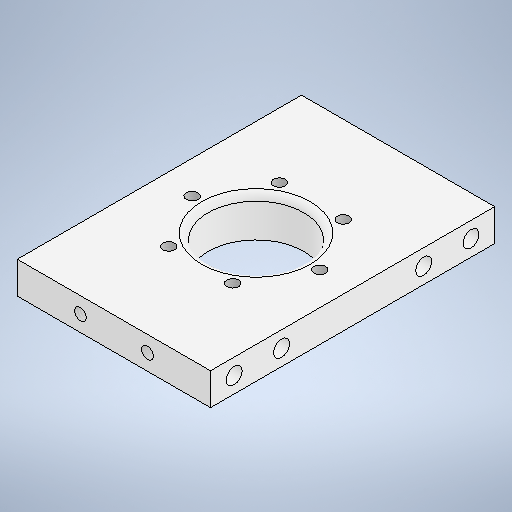
# Autodesk Inventor part: joint3_base2
Saved by Autodesk Inventor 2025.3 (Build 293356030, 356C)
## iProperties
Created: 2025-11-25
Part Number: joint3_base2
Material: PLA filament
Document SubType Name: Modeling
Designer: MSI
Mass: 55.5372 g
Surface Area: 164.624 cm^2
Volume: 46.281 cm^3
Density: 1.2 g/cm^3
Appearance: 일반
Author: MSI
Autodesk Inventor part; units mm, degrees
ref_plane "YZ Plane" through (0, 0, 0) normal (1, 0, 0) x (0, 1, 0)
ref_plane "XZ Plane" through (0, 0, 0) normal (0, 1, 0) x (-1, 0, 0)
ref_plane "XY Plane" through (0, 0, 0) normal (0, 0, 1) x (1, 0, 0)
sketch "스케치1" plane through (0, 0, 0) normal (0, 1, 0) x (-1, 0, 0)
  line L0 (107, -50) -> (-107, -50)
  line L1 (-107, -50) -> (-107, 50)
  line L2 (-107, 50) -> (107, 50)
  line L3 (107, 50) -> (107, -50)
  line L4 (107, -50) -> (-107, 50) construction
  line L5 (-107, -50) -> (107, 50) construction
  point P0 (0, 0)
  dimension "d0" = 214
  dimension "d1" = 100
  constraints: 12 end point, 2 midpoint, 2 parallel, 1 horizontal, 1 perpendicular
  measures "d0" distance of L1.end L2.end
  measures "d1" distance of L0.end L1.end
extrude "돌출1" add sketch "스케치1" along normal mid plane 10
sketch "스케치2" plane through (0, 5, 0) normal (0, 1, 0) x (1, 0, 0)
  point P0 (0, 0)
hole "구멍1" at (0, 5, 0) direction (0, -1, 0) diameter 30 end through all
fillet "모깎기2" radius 2 1 edges at (0, 5, -15)
sketch "스케치3" plane through (0, 5, 0) normal (0, 1, 0) x (1, 0, 0)
  line L0 (-107, 50) -> (-107, -50) projected
  line L1 (-107, 30) -> (-81.5, 30)
  line L2 (-81.5, 30) -> (-81.5, -30)
  line L3 (-81.5, -30) -> (-107, -30)
  line L4 (-107, -30) -> (-107, 30)
  line L5 (107, 50) -> (-107, 50) projected
  point P0 (0, 0)
  point P1 (-107, 0)
  dimension "d13" = 25.5
  dimension "d14" = 20
  constraints: 8 end point, 2 midpoint, 2 parallel, 1 horizontal, 1 perpendicular, 1 point on line
  measures "d13" distance of L2.end L3.end
  measures "d14" distance between parallel lines of L5 L1
extrude "돌출2" cut sketch "스케치3" against normal through all
sketch "스케치4" plane through (-81.5, 5, -30) normal (-1, 0, 0) x (0, 0, 1)
  line L0 (7, -5) -> (53, -5) construction
  point P0 (30, -5)
  point P1 (30, -5)
  point P2 (22.3333, -5)
  point P3 (37.6667, -5)
  dimension "d20" = 15.3333
  dimension "d21" = 15.3333
  dimension "d22" = 46
  constraints: 3 coincident, 2 end point, 2 point on line, 1 horizontal, 1 midpoint
  measures "d20" distance of point (22.333, -5) point (7, -5)
  measures "d21" distance of point (37.667, -5) point (53, -5)
  measures "d22" distance of L0.start L0.end
hole "구멍2" at (-81.5, 0, -23) at (-81.5, 0, -7.6667) at (-81.5, 0, 7.6667) at (-81.5, 0, 23) direction (1, 0, 0) diameter 3.6881 depth 12 tip angle 118 thread size "M4.5x0.75" class "6H" standard "ISO Metric profile"
sketch "스케치5" plane through (0, -5, 0) normal (0, -1, 0) x (1, 0, 0)
  line L0 (-100.75, -40) -> (-88.25, -40) construction
  line L1 (-88.25, -40) -> (-88.25, 40) construction
  line L2 (-88.25, 40) -> (-100.75, 40) construction
  line L3 (-100.75, 40) -> (-100.75, -40) construction
  line L4 (-107, -50) -> (107, -50) projected
  line L5 (-107, -30) -> (-107, -50) projected
  line L6 (107, 50) -> (-107, 50) projected
  point P0 (0, 0)
  dimension "d30" = 10
  dimension "d31" = 6.25
  dimension "d32" = 12.5
  dimension "d33" = 10
  constraints: 8 end point, 4 coincident, 2 parallel, 1 horizontal, 1 perpendicular
  measures "d30" distance between parallel lines of L0 L4
  measures "d31" distance between parallel lines of L3 L5
  measures "d32" distance of L0.start L0.end
  measures "d33" distance between parallel lines of L6 L2
hole "구멍3" at (-100.75, -5, -40) at (-88.25, -5, -40) at (-88.25, -5, 40) at (-100.75, -5, 40) direction (0, 1, 0) diameter 4.5 end through all counterbore diameter 8 counterbore depth 4.4 clearance for "Socket Head Cap Screw ISO 4762" size "M4" standard "ISO"
mirror "미러1" about plane through (0, 0, 0) normal (1, 0, 0) of "돌출2", "구멍2", "구멍3"
sketch "스케치6" plane through (0, -5, 0) normal (0, -1, 0) x (1, 0, 0)
  circle A0 centre (0, 0) radius 15 projected
  line L0 (25.9808, 0) -> (12.9904, -22.5)
  line L1 (12.9904, -22.5) -> (-12.9904, -22.5)
  line L2 (-12.9904, -22.5) -> (-25.9808, 0)
  line L3 (-25.9808, 0) -> (-12.9904, 22.5)
  line L4 (-12.9904, 22.5) -> (12.9904, 22.5)
  line L5 (12.9904, 22.5) -> (25.9808, 0)
  dimension "d41" = 45
  constraints: 12 end point, 1 coincident, 1 horizontal, 13 other
  measures "d41" distance between parallel lines of L1 L4
extrude "돌출3" add sketch "스케치6" along normal blind 2.5
sketch "스케치7" plane through (0, 5, 0) normal (0, 1, 0) x (1, 0, 0)
  line L0 (0, 0) -> (-20, 0) construction
  dimension "d44" = 20
  constraints: 2 end point, 1 horizontal
  measures "d44" distance of L0.start L0.end
hole "구멍4" at (-20, 5, 0) direction (0, -1, 0) diameter 3.6881 end through all thread size "M4.5x0.75" class "6H" standard "ISO Metric profile"
pattern_circular "원형 패턴1" count 6 over 360 about axis through (0, 3, 0) along (0, -1, 0) of "구멍4"
sketch "스케치8" plane through (0, -5, 0) normal (0, -1, 0) x (1, 0, 0)
  line L0 (-53.279, 16.5) -> (-38.279, 16.5) construction
  line L1 (-38.279, 16.5) -> (-38.279, -16.5) construction
  line L2 (-38.279, -16.5) -> (-53.279, -16.5) construction
  line L3 (-53.279, -16.5) -> (-53.279, 16.5) construction
  line L4 (-53.279, 16.5) -> (-38.279, -16.5) construction
  line L5 (-38.279, 16.5) -> (-53.279, -16.5) construction
  line L6 (-107, -50) -> (107, -50) projected
  line L7 (0, -50) -> (0, 50) construction
  line L8 (107, 50) -> (-107, 50) projected
  line L9 (-50.279, -13.5) -> (-41.279, -13.5) construction
  line L10 (-41.279, -13.5) -> (-41.279, 13.5) construction
  line L11 (-41.279, 13.5) -> (-50.279, 13.5) construction
  line L12 (-50.279, 13.5) -> (-50.279, -13.5) construction
  line L13 (53.279, 16.5) -> (38.279, 16.5) construction
  line L14 (38.279, 16.5) -> (38.279, -16.5) construction
  line L15 (38.279, -16.5) -> (53.279, -16.5) construction
  line L16 (53.279, -16.5) -> (53.279, 16.5) construction
  line L17 (53.279, 16.5) -> (38.279, -16.5) construction
  line L18 (38.279, 16.5) -> (53.279, -16.5) construction
  line L19 (50.279, -13.5) -> (41.279, -13.5) construction
  line L20 (41.279, -13.5) -> (41.279, 13.5) construction
  line L21 (41.279, 13.5) -> (50.279, 13.5) construction
  line L22 (50.279, 13.5) -> (50.279, -13.5) construction
  point P0 (0, 0)
  point P1 (-45.779, 0)
  point P2 (45.779, 0)
  dimension "d55" = 33
  dimension "d56" = 15
  dimension "d57" = 38.279
  dimension "d58" = 3
  constraints: 42 end point, 13 symmetric about line, 8 coincident, 4 midpoint, 4 parallel, 2 perpendicular, 1 horizontal, 1 horizontal alignment, 3 other
  measures "d55" distance of L2.end L0.start
  measures "d56" distance of L1.end L2.end
  measures "d57" distance between parallel lines of L7 L1
  measures "d58" distance between parallel lines of L2 L9
hole "구멍5" at (-50.279, -5, 13.5) at (-41.279, -5, 13.5) at (-41.279, -5, -13.5) at (-50.279, -5, -13.5) at (50.279, -5, -13.5) at (41.279, -5, -13.5) at (41.279, -5, 13.5) at (50.279, -5, 13.5) direction (0, 1, 0) diameter 4.5 end through all counterbore diameter 8 counterbore depth 4.6 clearance for "Socket Head Cap Screw ISO 4762" size "M4" standard "ISO"
chamfer "모따기1" distance 1 angle 45 4 edges at (107, 0, -30) (107, 0, 30) (-107, 0, -30) (-107, 0, 30)
fillet "모깎기1" radius 3 10 edges at (107, 0, 50) (107, 0, -50) (-107, 0, -50) (-107, 0, 50) (-12.9904, -6.25, -22.5) (12.9904, -6.25, 22.5) (-12.9904, -6.25, 22.5) (-25.9808, -6.25, 0) (25.9808, -6.25, 0) (12.9904, -6.25, -22.5)
sketch "스케치9" plane through (-104, -5, 50) normal (0, 0, 1) x (1, 0, 0)
  line L0 (208, 10) -> (0, 10) projected
  line L1 (0, 0) -> (208, 0) projected
  line L2 (43, 10) -> (104, 10)
  line L3 (104, 10) -> (104, 0)
  line L4 (104, 0) -> (43, 0)
  line L5 (43, 0) -> (43, 10)
  point P0 (104, 5)
  point P1 (73.5, 10)
  point P2 (43, 0)
  dimension "d66" = 30.5
  dimension "d67" = 61
  constraints: 8 end point, 2 midpoint, 2 parallel, 1 horizontal, 1 perpendicular, 1 point on line
  measures "d66" horizontal distance of point (104, 5) point (73.5, 10)
  measures "d67" distance between parallel lines of L3 L5
extrude "돌출4" cut sketch "스케치9" against normal blind 5.5
sketch "스케치10" plane through (-104, -5, 44.5) normal (0, 0, 1) x (1, 0, 0)
  line L0 (53.5, 5) -> (93.5, 5) construction
  line L1 (43, 10) -> (104, 10) projected
  line L2 (104, 10) -> (104, 0) projected
  point P0 (104, 5)
  point P1 (73.5, 5)
  point P2 (73.5, 10)
  point P3 (104, 5)
  dimension "d70" = 40
  constraints: 3 midpoint, 2 coincident, 2 end point, 1 horizontal, 1 point on line, 1 vertical alignment
  measures "d70" distance of L0.start L0.end
hole "구멍6" at (-50.5, 0, 44.5) at (-10.5, 0, 44.5) direction (0, 0, -1) diameter 3.6881 depth 13 tip angle 118 thread size "M4.5x0.75" class "6H" standard "ISO Metric profile"
mirror "미러2" about plane through (0, 0, 0) normal (0, 0, 1) of "구멍6", "돌출4"
mirror "미러3" about plane through (0, 0, 0) normal (1, 0, 0) of "구멍6", "돌출4", "미러2"
chamfer "모따기2" distance 1 angle 45 4 edges at (-61, 0, 50) (61, 0, 50) (-61, 0, -50) (61, 0, -50)
sketch "스케치11" plane through (0, 5, 0) normal (0, 1, 0) x (1, 0, 0)
  line L0 (-61, 44.5) -> (61, 44.5) projected
  line L1 (-30.5, 44.5) -> (-30.5, -44.5) construction
  line L2 (61, -44.5) -> (-61, -44.5) projected
  line L3 (-30.25, 79.6177) -> (30.25, 79.6177)
  line L4 (30.25, 79.6177) -> (30.25, -99.7014)
  line L5 (30.25, -99.7014) -> (-30.25, -99.7014)
  line L6 (-30.25, -99.7014) -> (-30.25, 79.6177)
  line L7 (30.5, -44.5) -> (30.5, 44.5) construction
  point P0 (0, 0)
  dimension "d81" = 30.5
  dimension "d95" = 30.5
  dimension "d96" = 0.25
  dimension "d97" = 0.25
  constraints: 12 end point, 4 point on line, 2 parallel, 2 perpendicular, 1 horizontal, 1 vertical
  measures "d81" distance from line of point (0, 0) L1
  measures "d95" distance from line of L7 point (0, 0)
  measures "d96" distance between parallel lines of L1 L6
  measures "d97" distance between parallel lines of L4 L7
extrude "돌출5" cut sketch "스케치11" against normal through all keep common part
sketch "스케치12" plane through (-30.25, 5, 44.5) normal (-1, 0, 0) x (0, 0, 1)
  line L0 (-81.5833, -5) -> (-7.4167, -5) construction
  point P0 (-44.5, -5)
  point P1 (-44.5, -5)
  point P2 (-66.75, -5)
  point P3 (-22.25, -5)
  dimension "d85" = 14.8333
  dimension "d86" = 14.8333
  dimension "d87" = 74.1667
  constraints: 3 coincident, 2 end point, 2 point on line, 1 horizontal, 1 midpoint
  measures "d85" distance of point (-66.75, -5) L0.start
  measures "d86" distance of point (-22.25, -5) point (-7.417, -5)
  measures "d87" distance of L0.start L0.end
hole "구멍7" at (-30.25, 0, -37.0833) at (-30.25, 0, -22.25) at (-30.25, 0, 22.25) at (-30.25, 0, 37.0833) direction (1, 0, 0) diameter 5 depth 10 tip angle 118
mirror "미러4" about plane through (0, 0, 0) normal (1, 0, 0) of "구멍7"
equation "\"d21\" = d20"
equation "\"d22\" = 3 * d20"
equation "\"d31\" = 0.5 * d32"
equation "\"d33\" = d30"
equation "\"d95\" = d81"
equation "\"d97\" = d96"
equation "\"d86\" = d85"
equation "\"d87\" = 5 * d85"
